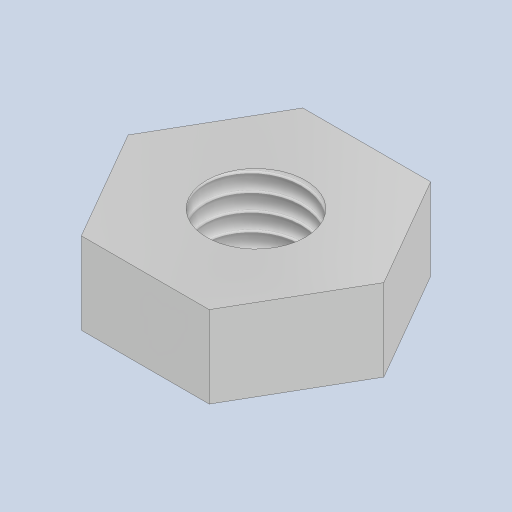
# Autodesk Inventor part: Porca 2,9mm
Saved by Autodesk Inventor 2024.3 (Build 283343000, 343)
## iProperties
Created: 2025-01-14
Part Number: Porca 2,9mm
Material: Aço
Document SubType Name: Modeling
Designer: Cliente
Density: 7.85 g/cm^3
Appearance: Placa
Mass: 0.564906 g
Surface Area: 1.35874 cm^2
Volume: 0.0719625 cm^3
Author: Cliente
Autodesk Inventor part; units mm, degrees
ref_plane "YZ Plane" through (0, 0, 0) normal (1, 0, 0) x (0, 1, 0)
ref_plane "XZ Plane" through (0, 0, 0) normal (0, 1, 0) x (-1, 0, 0)
ref_plane "XY Plane" through (0, 0, 0) normal (0, 0, 1) x (1, 0, 0)
sketch "Esboço1" plane through (0, 0, 0) normal (0, 1, 0) x (-1, 0, 0)
  line L0 (3.7528, 0) -> (1.8764, -3.25)
  line L1 (1.8764, -3.25) -> (-1.8764, -3.25)
  line L2 (-1.8764, -3.25) -> (-3.7528, 0)
  line L3 (-3.7528, 0) -> (-1.8764, 3.25)
  line L4 (-1.8764, 3.25) -> (1.8764, 3.25)
  line L5 (1.8764, 3.25) -> (3.7528, 0)
  circle A0 centre (0, 0) radius 1.45
  dimension "d0" = 6.5
  dimension "d1" = 2.9
  constraints: 12 end point, 2 coincident, 1 centre point, 1 horizontal alignment, 13 other
  measures "d0" distance between parallel lines of L4 L1
  measures "d1" diameter of A0
extrude "Extrusão1" add sketch "Esboço1" along normal blind 2.4
thread "Rosca1" size "M3x0.5" class "6H" standard "ANSI Metric M Profile" full length
